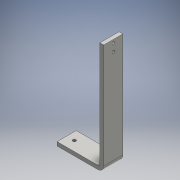
# Autodesk Inventor part: Brazo
Saved by Autodesk Inventor 2016 (Build 200138000, 138)
## iProperties
Created: 2016-04-04
Part Number: Brazo
Material: Generic
Document SubType Name: Modeling
Designer: Andres
Density: 1 g/cm^3
Appearance: Default
Author: Andres
Autodesk Inventor part; units mm, degrees
ref_plane "YZ Plane" through (0, 0, 0) normal (1, 0, 0) x (0, 1, 0)
ref_plane "XZ Plane" through (0, 0, 0) normal (0, 1, 0) x (-1, 0, 0)
ref_plane "XY Plane" through (0, 0, 0) normal (0, 0, 1) x (1, 0, 0)
sketch "Sketch1" plane through (0, 0, 0) normal (0, 1, 0) x (-1, 0, 0)
  line L0 (0, 0) -> (0, -137)
  line L1 (3, -140) -> (56, -140)
  arc A0 (0, -137) -> (3, -140) centre (3, -137) ccw
  line L2 (56, -145) -> (3, -145)
  arc A1 (-5, -137) -> (3, -145) centre (3, -137) ccw
  line L3 (-5, -137) -> (-5, 0)
  line L4 (56, -140) -> (56, -145)
  line L5 (-5, 0) -> (0, 0)
  point P0 (0, -140)
  dimension "d0" = 140
  dimension "d1" = 56
  dimension "d2" = 3
  dimension "d3" = 5
  constraints: 12 end point, 4 point on circle, 3 perpendicular, 2 centre point, 2 point on line, 2 tangent, 2 vertical, 2 other
  measures "d0" distance of L0.start point (0, -140)
  measures "d1" distance of point (0, -140) L1.end
  measures "d2" radius of A0
  measures "d3" distance between parallel lines of L1 L2
extrude "Extrusion1" add sketch "Sketch1" along normal blind 25
sketch "Sketch2" plane through (-3, 0, -145) normal (0, 0, -1) x (-1, 0, 0)
  line L0 (53, 0) -> (0, 0) projected
  line L1 (53, 0) -> (53, 25) projected
  line L2 (0, 25) -> (53, 25) projected
  line L3 (0, 0) -> (0, 25) projected
  circle A0 centre (43, 12.5) radius 2
  point P0 (-3, 0)
  dimension "d6" = 4
  dimension "d7" = 12.5
  dimension "d8" = 10
  constraints: 1 centre point
  measures "d6" diameter of A0
  measures "d7" distance from line of L2 A0.centre
  measures "d8" distance from line of L1 A0.centre
hole "Hole1" at (-46, 12.5, -145) direction (0, 0, 1) diameter 4 end through all
sketch "Sketch3" plane through (0, 0, -137) normal (-1, 0, 0) x (0, 0, 1)
  line L0 (137, 0) -> (0, 0) projected
  line L1 (137, 0) -> (137, 25) projected
  line L2 (0, 25) -> (137, 25) projected
  line L3 (0, 0) -> (0, 25) projected
  circle A0 centre (123, 12.5) radius 2
  circle A1 centre (133, 12.5) radius 2
  dimension "d16" = 4
  dimension "d17" = 4
  dimension "d18" = 4
  dimension "d19" = 14
  dimension "d20" = 12.5
  dimension "d21" = 12.5
  constraints: 2 centre point
  measures "d16" diameter of A0
  measures "d17" diameter of A1
  measures "d18" distance from line of L1 A1.centre
  measures "d19" distance from line of L1 A0.centre
  measures "d20" distance from line of L2 A1.centre
  measures "d21" distance from line of L2 A0.centre
hole "Hole2" at (0, 12.5, -14) at (0, 12.5, -4) direction (1, 0, 0) diameter 3.302 end through all
body "Solid1"
